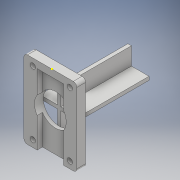
# Autodesk Inventor part: drzakfotorezistoru
Saved by Autodesk Inventor 2017 (Build 210142000, 142)
## iProperties
Created: 2019-02-02
Part Number: drzakfotorezistoru
Material: Generic
Document SubType Name: Modeling
Designer: Denis Kurka
Density: 1 g/cm^3
Appearance: Default
Author: Denis Kurka
Autodesk Inventor part; units mm, degrees
ref_plane "YZ Plane" through (0, 0, 0) normal (1, 0, 0) x (0, 1, 0)
ref_plane "XZ Plane" through (0, 0, 0) normal (0, 1, 0) x (-1, 0, 0)
ref_plane "XY Plane" through (0, 0, 0) normal (0, 0, 1) x (1, 0, 0)
sketch "Sketch1" plane through (0, 0, 0) normal (0, 1, 0) x (-1, 0, 0)
  line L0 (0, 0) -> (30, 0)
  line L1 (30, 0) -> (30, -44)
  line L2 (30, -44) -> (0, -44)
  line L3 (0, -44) -> (0, 0)
  circle A0 centre (24.9, -3.9) radius 1.5
  circle A1 centre (3.9, -3.9) radius 1.5
  circle A2 centre (3.9, -40.1) radius 1.5
  circle A3 centre (24.9, -40.1) radius 1.5
  circle A4 centre (15, -22) radius 9
  dimension "d0" = 44
  dimension "d1" = 30
  dimension "d2" = 3
  dimension "d3" = 3
  dimension "d4" = 3
  dimension "d5" = 3
  dimension "d8" = 3.9
  dimension "d9" = 3.9
  dimension "d10" = 3.9
  dimension "d11" = 3.9
  dimension "d12" = 3.9
  dimension "d14" = 21
  dimension "d15" = 3.9
  dimension "d17" = 21
  dimension "d18" = 18
  dimension "d19" = 22
  dimension "d20" = 15
  constraints: 8 end point, 5 centre point, 2 parallel, 1 horizontal, 1 perpendicular
  measures "d0" distance of L0.end L1.end
  measures "d1" distance of L1.end L2.end
  measures "d2" diameter of A0
  measures "d3" diameter of A1
  measures "d4" diameter of A2
  measures "d5" diameter of A3
  measures "d8" distance from line of L0 A0.centre
  measures "d9" distance from line of L0 A1.centre
  measures "d10" distance from line of L3 A1.centre
  measures "d11" distance from line of L2 A2.centre
  measures "d12" distance from line of L3 A2.centre
  measures "d14" distance of A1.centre A0.centre
  measures "d15" distance from line of L2 A3.centre
  measures "d17" distance of A2.centre A3.centre
  measures "d18" diameter of A4
  measures "d19" distance from line of L0 A4.centre
  measures "d20" distance from line of L1 A4.centre
extrude "Extrusion1" add sketch "Sketch1" along normal blind 5
sketch "Sketch2" plane through (0, 0, 0) normal (0, -1, 0) x (1, 0, 0)
  line L0 (-7.5, -44) -> (-22.5, -44)
  line L1 (-22.5, -44) -> (-22.5, -4)
  line L2 (-22.5, -4) -> (-7.5, -4)
  line L3 (-7.5, -4) -> (-7.5, -44)
  line L4 (0, 0) -> (-30, 0) projected
  line L5 (-30, -44) -> (0, -44) projected
  line L6 (0, -44) -> (0, 0) projected
  line L7 (-30, 0) -> (-30, -44) projected
  dimension "d24" = 4
  dimension "d25" = 0
  dimension "d26" = 15
  dimension "d27" = 7.5
  dimension "d28" = 7.5
  constraints: 8 end point, 2 parallel, 1 horizontal, 1 perpendicular
  measures "d24" distance between parallel lines of L2 L4
  measures "d25" distance between parallel lines of L5 L0
  measures "d26" distance between parallel lines of L1 L3
  measures "d27" distance between parallel lines of L6 L3
  measures "d28" distance between parallel lines of L7 L1
extrude "Extrusion2" cut sketch "Sketch2" against normal blind 3 contours L0 L1 L2 L3
fillet "Fillet1" radius 2 4 edges at (0, 2.5, 0) (-30, 2.5, 0) (-30, 2.5, -44) (0, 2.5, -44)
sketch "Sketch3" plane through (0, 5, 0) normal (0, 1, 0) x (1, 0, 0)
  line L0 (-26, 23) -> (-4, 23)
  line L1 (-4, 23) -> (-4, 21)
  line L2 (-4, 21) -> (-26, 21)
  line L3 (-26, 21) -> (-26, 23)
  line L4 (-2, 44) -> (-28, 44) projected
  circle A0 centre (-15, 22) radius 9 projected
  line L5 (-16, 33) -> (-14, 33)
  line L6 (-14, 33) -> (-14, 11)
  line L7 (-14, 11) -> (-16, 11)
  line L8 (-16, 11) -> (-16, 33)
  line L9 (-30, 42) -> (-30, 2) projected
  point P0 (0, 0)
  dimension "d32" = 2
  dimension "d33" = 21
  dimension "d34" = 11
  dimension "d35" = 11
  dimension "d36" = 14
  dimension "d37" = 2
  dimension "d38" = 11
  dimension "d39" = 11
  constraints: 16 end point, 4 parallel, 2 horizontal, 2 perpendicular
  measures "d32" distance of L2.end L0.start
  measures "d33" distance between parallel lines of L4 L0
  measures "d34" distance from line of A0.centre L3
  measures "d35" distance from line of A0.centre L1
  measures "d36" distance between parallel lines of L9 L8
  measures "d37" distance of L6.end L7.end
  measures "d38" distance from line of A0.centre L7
  measures "d39" distance from line of A0.centre L5
extrude "Extrusion3" add sketch "Sketch3" along normal blind 40 contours L0 A0 L2 L3 | L0 L8 L2 A0 | L8 A0 L6 L0 | L0 L6 L2 L8 | L8 L5 L6 A0 | L0 A0 L2 L6 | L2 L6 A0 L8 | A0 L6 L7 L8 | L0 L1 L2 A0
sketch "Sketch4" plane through (-14, 5, -13.0557) normal (1, 0, 0) x (0, 0, -1)
  point P0 (-13.0557, -5)
body "Solid1"
